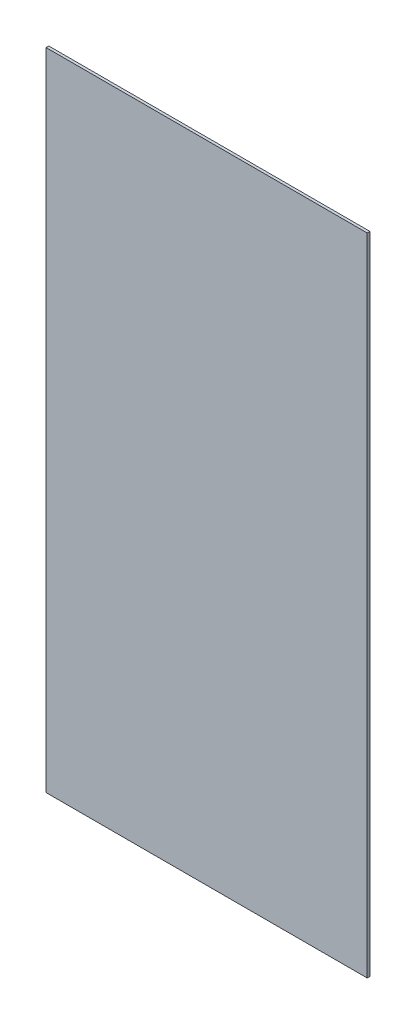
# Autodesk Inventor part: solar cell 26x52
Saved by Autodesk Inventor 2017 (Build 210142000, 142)
## iProperties
Created: 2017-04-29
Part Number: solar cell 26x52
Material: Generic
Document SubType Name: Modeling
Designer: X220T
Density: 1 g/cm^3
Appearance: Default
Author: X220T
Autodesk Inventor part; units mm, degrees
ref_plane "YZ Plane" through (0, 0, 0) normal (1, 0, 0) x (0, 1, 0)
ref_plane "XZ Plane" through (0, 0, 0) normal (0, 1, 0) x (-1, 0, 0)
ref_plane "XY Plane" through (0, 0, 0) normal (0, 0, 1) x (1, 0, 0)
sketch "Sketch1" plane through (0, 0, 0) normal (0, 0, 1) x (1, 0, 0)
  line L0 (-13, -26.125) -> (13, -26.125)
  line L1 (13, -26.125) -> (13, 26.125)
  line L2 (13, 26.125) -> (-13, 26.125)
  line L3 (-13, 26.125) -> (-13, -26.125)
  line L4 (-13, -26.125) -> (13, 26.125) construction
  line L5 (13, -26.125) -> (-13, 26.125) construction
  point P0 (0, 0)
  dimension "d0" = 26
  dimension "d1" = 52.25
  constraints: 12 end point, 2 midpoint, 2 parallel, 1 horizontal, 1 perpendicular
  measures "d0" distance of L2.end L1.end
  measures "d1" distance of L1.end L0.end
extrude "Extrusion1" add sketch "Sketch1" along normal blind 0.22
body "Solid1"
